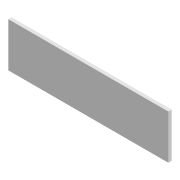
# Autodesk Inventor part: 00_Baseplate_Simmo_side4_v2
Saved by Autodesk Inventor 2022 (Build 260153000, 153)
## iProperties
Created: 2022-08-04
Part Number: 00_Baseplate_Simmo_side4_v2
Material: Generic
Document SubType Name: Modeling
Designer: wanghaoran
Density: 1 g/cm^3
Appearance: Default
Author: wanghaoran
Autodesk Inventor part; units mm, degrees
ref_plane "YZ Plane" through (0, 0, 0) normal (1, 0, 0) x (0, 1, 0)
ref_plane "XZ Plane" through (0, 0, 0) normal (0, 1, 0) x (-1, 0, 0)
ref_plane "XY Plane" through (0, 0, 0) normal (0, 0, 1) x (1, 0, 0)
sketch "Sketch1" plane through (0, 0, 0) normal (0, 0, 1) x (1, 0, 0)
  line L0 (15.4242, 6) -> (15.4242, -73) projected
  line L1 (-270, 0) -> (-270, 6) projected
  line L2 (15.4242, 6) -> (-270, 6)
  line L3 (-270, 6) -> (-270, -73)
  line L4 (-270, -73) -> (15.4242, -73)
  line L5 (15.4242, -73) -> (15.4242, 6)
  line L6 (-276, 0) -> (-276, 6) projected
  line L7 (-270, 6) -> (-276, 6)
  line L8 (-276, 6) -> (-276, -73)
  line L9 (-276, -73) -> (-270, -73)
  line L10 (-270, -73) -> (-270, 6)
  point P0 (0, 0)
  dimension "d0" = 79
  constraints: 16 end point, 4 parallel, 2 horizontal, 2 perpendicular
  measures "d0" distance of L3.end L2.end
extrude "Extrusion1" add sketch "Sketch1" along normal blind 6
sketch "Sketch2" plane through (0, 0, 6) normal (0, 0, 1) x (1, 0, 0)
  line L0 (0, 0) -> (0, 6) projected
  line L1 (15.4242, 6) -> (-276, 6) projected
  line L2 (0, 0) -> (15.4242, 0)
  line L3 (15.4242, -73) -> (15.4242, 6) projected
  line L4 (0, 6) -> (-0.1, 6)
  line L5 (-0.1, 6) -> (-0.1, 0)
  line L6 (-0.1, 0) -> (0, 0)
  line L7 (0, 0) -> (0, 6)
  point P0 (-270, 6)
  dimension "d5" = 0.1
  constraints: 10 end point, 2 horizontal, 2 parallel, 1 perpendicular, 1 point on line
  measures "d5" distance of L6.end L5.end
extrude "Extrusion2" cut sketch "Sketch2" against normal blind 6
sketch "Sketch3" plane through (0, 0, 6) normal (0, 0, 1) x (1, 0, 0)
  line L0 (-10, 0) -> (-10, 6) projected
  line L1 (-20, 6) -> (-10, 6) projected
  line L2 (-20, 6) -> (-20, 0) projected
  line L3 (-20, 0) -> (-10, 0) projected
  line L4 (-0.1, 6) -> (-276, 6) projected
  line L5 (-10, 0) -> (-9.9, 0)
  line L6 (-9.9, 0) -> (-9.9, 6)
  line L7 (-9.9, 6) -> (-10, 6)
  line L8 (-10, 6) -> (-10, 0)
  line L9 (-20, 0) -> (-20.1, 0)
  line L10 (-20.1, 0) -> (-20.1, 6)
  line L11 (-20.1, 6) -> (-20, 6)
  line L12 (-20, 6) -> (-20, 0)
  point P0 (0, 0)
  point P1 (-270, 6)
  dimension "d6" = 0.1
  dimension "d7" = 0.1
  constraints: 16 end point, 4 parallel, 2 horizontal, 2 perpendicular, 2 point on line
  measures "d6" distance of L7.end L6.end
  measures "d7" distance of L10.end L11.end
extrude "Extrusion3" cut sketch "Sketch3" against normal blind 6
pattern_linear "Rectangular Pattern1" count 13 spacing 20 along (-1, 0, 0) of "Extrusion3"
ref_plane "Work Plane1" through (-276, -33.5, 6) normal (0, 1, 0) x (1, 0, 0)
sketch "Sketch4" plane through (0, 0, 6) normal (0, 0, 1) x (1, 0, 0)
  line L0 (-260.1, 0) -> (-260.1, 6) projected
  line L1 (-249.9, 6) -> (-249.9, 0) projected
  line L2 (-334.2848, -33.5) -> (73.709, -33.5) projected
  line L3 (-260.1, -67) -> (-260.1, -73)
  line L4 (-249.9, -73) -> (-249.9, -67)
  line L5 (-249.9, -67) -> (-260.1, -67)
  line L6 (-276, -73) -> (15.4242, -73) projected
  point P0 (0, 0)
  constraints: 6 end point, 4 symmetric about line, 1 horizontal
extrude "Extrusion4" cut sketch "Sketch4" against normal blind 6
pattern_linear "Rectangular Pattern2" count 14 spacing 20 along (1, 0, 0) of "Extrusion4"
body "Solid1"
